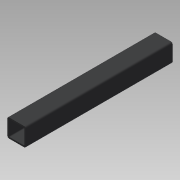
# Autodesk Inventor part: 9700
Saved by Autodesk Inventor 2013 (Build 170138000, 138)
## iProperties
Company: 80/20 Inc.
Created: 2014-04-23
Part Number: 9700
Material: Generic
Document SubType Name: Modeling
Density: 1 g/cm^3
Vendor: 80/20 Inc.
Engineer: Ross Bowman
Designer: Ross Bowman
Catalog Web Link: 8020.net
Material: 6105-T5 Aluminum
Author: Ross Bowman
Keywords: 80/20 , 8020 , T-Slot , Extrusion
Autodesk Inventor part; units mm, degrees
ref_plane "YZ Plane" through (0, 0, 0) normal (1, 0, 0) x (0, 1, 0)
ref_plane "XZ Plane" through (0, 0, 0) normal (0, 1, 0) x (-1, 0, 0)
ref_plane "XY Plane" through (0, 0, 0) normal (0, 0, 1) x (1, 0, 0)
sketch "Sketch1" plane through (0, 0, 0) normal (0, 0, 1) x (1, 0, 0)
  line L0 (-15.875, 14.2748) -> (-15.875, -14.2748)
  arc A0 (-14.2748, 15.875) -> (-15.875, 14.2748) centre (-14.2748, 14.2748) ccw
  line L1 (14.2748, 15.875) -> (-14.2748, 15.875)
  arc A1 (15.875, 14.2748) -> (14.2748, 15.875) centre (14.2748, 14.2748) ccw
  line L2 (15.875, -14.2748) -> (15.875, 14.2748)
  arc A2 (14.2748, -15.875) -> (15.875, -14.2748) centre (14.2748, -14.2748) ccw
  line L3 (-14.2748, -15.875) -> (14.2748, -15.875)
  arc A3 (-15.875, -14.2748) -> (-14.2748, -15.875) centre (-14.2748, -14.2748) ccw
  arc A4 (19.05, 15.875) -> (15.875, 19.05) centre (15.875, 15.875) ccw
  line L4 (15.875, 19.05) -> (-15.875, 19.05)
  arc A5 (-15.875, 19.05) -> (-19.05, 15.875) centre (-15.875, 15.875) ccw
  line L5 (-19.05, 15.875) -> (-19.05, -15.875)
  arc A6 (-19.05, -15.875) -> (-15.875, -19.05) centre (-15.875, -15.875) ccw
  line L6 (-15.875, -19.05) -> (15.875, -19.05)
  arc A7 (15.875, -19.05) -> (19.05, -15.875) centre (15.875, -15.875) ccw
  line L7 (19.05, -15.875) -> (19.05, 15.875)
  point P0 (0, 0)
  constraints: 16 end point, 16 point on circle, 8 centre point
extrude "Extrusion1" add sketch "Sketch1" against normal blind 304.8
body "Solid1"
